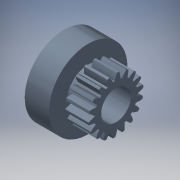
# Autodesk Inventor part: Clutch Gear
Saved by Autodesk Inventor 2019 Beta2 (Build 230110000, 110) ContinuousBuild 0
## iProperties
Created: 2012-08-06
Part Number: Clutch Gear
Material: Stainless Steel, 440C
Document SubType Name: Modeling
Designer: John
Density: 7.75 g/cm^3
Mass: 13.9161 g
Surface Area: 27.6405 cm^2
Volume: 1.79562 cm^3
Appearance: Steel Blue
Author: John
Autodesk Inventor part; units mm, degrees
ref_plane "YZ Plane" through (0, 0, 0) normal (1, 0, 0) x (0, 1, 0)
ref_plane "XZ Plane" through (0, 0, 0) normal (0, 1, 0) x (-1, 0, 0)
ref_plane "XY Plane" through (0, 0, 0) normal (0, 0, 1) x (1, 0, 0)
sketch "Sketch1" plane through (0, 0, 0) normal (1, 0, 0) x (0, 1, 0)
  circle A0 centre (0, 0) radius 12.5095
  dimension "d0" = 25.019
  constraints: 1 centre point, 1 coincident
  measures "d0" diameter of A0
extrude "Extrusion1" add sketch "Sketch1" along normal blind 7.747
sketch "Sketch3" plane through (7.747, 0, 0) normal (1, 0, 0) x (0, 0, -1)
  circle A0 centre (0, 0) radius 12.5095 projected
  circle A1 centre (0, 0) radius 8.763
  dimension "d3" = 17.526
  constraints: 1 centre point, 1 coincident
  measures "d3" diameter of A1
extrude "Extrusion2" add sketch "Sketch3" along normal blind 8.89 contours A1
sketch "Sketch4" plane through (7.747, 0, 0) normal (1, 0, 0) x (0, 0, -1)
  circle A0 centre (0, 0) radius 8.763 projected
  circle A1 centre (0, 0) radius 6.7818
  dimension "d26" = 6.7818
  constraints: 1 centre point
  measures "d26" radius of A1
extrude "Extrusion3" cut sketch "Sketch4" along normal blind 1.397
sketch "Sketch5" plane through (16.637, 0, 0) normal (1, 0, 0) x (0, 0, -1)
  circle A0 centre (0, 0) radius 8.763 projected
hole "Hole1" at (16.637, 0, 0) direction (-1, 0, 0) diameter 9.525 end through all
sketch "Sketch6" plane through (0, 0, 0) normal (-1, 0, 0) x (0, 0, 1)
  circle A0 centre (0, 0) radius 4.7625 projected
hole "Hole2" at (0, 0, 0) direction (1, 0, 0) diameter 23.114 depth 6.8072
sketch "Sketch7" plane through (16.637, 0, 0) normal (1, 0, 0) x (0, 0, -1)
  circle A0 centre (0, 0) radius 8.763 projected
  arc A1 (6.3049, -2.5147) -> (8.3872, -2.5234) centre (7.3744, 4.2693) ccw
  arc A2 (8.3872, -2.5234) -> (8.5753, -1.7828) centre (0, 0) ccw
  arc A3 (8.5753, -1.7828) -> (6.741, -0.7972) centre (4.445, -7.2699) ccw
  arc A4 (6.741, -0.7972) -> (6.7848, -0.2067) centre (0, 0) ccw
  arc A5 (6.7848, -0.2067) -> (8.7445, 0.4974) centre (5.4695, 6.534) ccw
  arc A6 (8.7445, 0.4974) -> (8.6679, 1.2576) centre (0, 0) ccw
  arc A7 (8.6679, 1.2576) -> (6.6071, 1.5564) centre (6.6633, -5.3112) ccw
  arc A8 (6.6071, 1.5564) -> (6.4463, 2.1263) centre (0, 0) ccw
  arc A9 (6.4463, 2.1263) -> (8.047, 3.4581) centre (2.9049, 8.0107) ccw
  arc A10 (8.047, 3.4581) -> (7.715, 4.1463) centre (0, 0) ccw
  arc A11 (7.715, 4.1463) -> (5.6763, 3.7223) centre (8.078, -2.7119) ccw
  arc A12 (5.6763, 3.7223) -> (5.3303, 4.2029) centre (0, 0) ccw
  arc A13 (5.3303, 4.2029) -> (6.379, 6.0018) centre (-0.0101, 8.5211) ccw
  arc A14 (6.379, 6.0018) -> (5.8316, 6.535) centre (0, 0) ccw
  arc A15 (5.8316, 6.535) -> (4.0609, 5.4392) centre (8.5184, 0.2145) ccw
  arc A16 (4.0609, 5.4392) -> (3.5714, 5.7725) centre (0, 0) ccw
  arc A17 (3.5714, 5.7725) -> (3.9415, 7.8216) centre (-2.9239, 8.0037) ccw
  arc A18 (3.9415, 7.8216) -> (3.2448, 8.1354) centre (0, 0) ccw
  arc A19 (3.2448, 8.1354) -> (1.9557, 6.5001) centre (7.9313, 3.115) ccw
  arc A20 (1.9557, 6.5001) -> (1.3817, 6.6458) centre (0, 0) ccw
  arc A21 (1.3817, 6.6458) -> (1.0287, 8.698) centre (-5.485, 6.521) ccw
  arc A22 (1.0287, 8.698) -> (0.2667, 8.7546) centre (0, 0) ccw
  arc A23 (0.2667, 8.7546) -> (-0.3854, 6.777) centre (6.3876, 5.6398) ccw
  arc A24 (-0.3854, 6.777) -> (-0.9746, 6.7176) centre (0, 0) ccw
  arc A25 (-0.9746, 6.7176) -> (-2.0083, 8.5253) centre (-7.3845, 4.2518) ccw
  arc A26 (-2.0083, 8.5253) -> (-2.7436, 8.3178) centre (0, 0) ccw
  arc A27 (-2.7436, 8.3178) -> (-2.6801, 6.2364) centre (4.0734, 7.4844) ccw
  arc A28 (-2.6801, 6.2364) -> (-3.2134, 5.9791) centre (0, 0) ccw
  arc A29 (-3.2134, 5.9791) -> (-4.803, 7.3243) centre (-8.3934, 1.4697) ccw
  arc A30 (-4.803, 7.3243) -> (-5.423, 6.8778) centre (0, 0) ccw
  arc A31 (-5.423, 6.8778) -> (-4.6514, 4.9437) centre (1.268, 8.4262) ccw
  arc A32 (-4.6514, 4.9437) -> (-5.0646, 4.5195) centre (0, 0) ccw
  arc A33 (-5.0646, 4.5195) -> (-7.0184, 5.2399) centre (-8.3899, -1.4896) ccw
  arc A34 (-7.0184, 5.2399) -> (-7.4483, 4.6082) centre (0, 0) ccw
  arc A35 (-7.4483, 4.6082) -> (-6.0618, 3.0547) centre (-1.6904, 8.3517) ccw
  arc A36 (-6.0618, 3.0547) -> (-6.3049, 2.5147) centre (0, 0) ccw
  arc A37 (-6.3049, 2.5147) -> (-8.3872, 2.5234) centre (-7.3744, -4.2693) ccw
  arc A38 (-8.3872, 2.5234) -> (-8.5753, 1.7828) centre (0, 0) ccw
  arc A39 (-8.5753, 1.7828) -> (-6.741, 0.7972) centre (-4.445, 7.2699) ccw
  arc A40 (-6.741, 0.7972) -> (-6.7848, 0.2067) centre (0, 0) ccw
  arc A41 (-6.7848, 0.2067) -> (-8.7445, -0.4974) centre (-5.4695, -6.534) ccw
  arc A42 (-8.7445, -0.4974) -> (-8.6679, -1.2576) centre (0, 0) ccw
  arc A43 (-8.6679, -1.2576) -> (-6.6071, -1.5564) centre (-6.6633, 5.3112) ccw
  arc A44 (-6.6071, -1.5564) -> (-6.4463, -2.1263) centre (0, 0) ccw
  arc A45 (-6.4463, -2.1263) -> (-8.047, -3.4581) centre (-2.9049, -8.0107) ccw
  arc A46 (-8.047, -3.4581) -> (-7.715, -4.1463) centre (0, 0) ccw
  arc A47 (-7.715, -4.1463) -> (-5.6763, -3.7223) centre (-8.078, 2.7119) ccw
  arc A48 (-5.6763, -3.7223) -> (-5.3303, -4.2029) centre (0, 0) ccw
  arc A49 (-5.3303, -4.2029) -> (-6.379, -6.0018) centre (0.0101, -8.5211) ccw
  arc A50 (-6.379, -6.0018) -> (-5.8316, -6.535) centre (0, 0) ccw
  arc A51 (-5.8316, -6.535) -> (-4.0609, -5.4392) centre (-8.5184, -0.2145) ccw
  arc A52 (-4.0609, -5.4392) -> (-3.5714, -5.7725) centre (0, 0) ccw
  arc A53 (-3.5714, -5.7725) -> (-3.9415, -7.8216) centre (2.9239, -8.0037) ccw
  arc A54 (-3.9415, -7.8216) -> (-3.2448, -8.1354) centre (0, 0) ccw
  arc A55 (-3.2448, -8.1354) -> (-1.9557, -6.5001) centre (-7.9313, -3.115) ccw
  arc A56 (-1.9557, -6.5001) -> (-1.3817, -6.6458) centre (0, 0) ccw
  arc A57 (-1.3817, -6.6458) -> (-1.0287, -8.698) centre (5.485, -6.521) ccw
  arc A58 (-1.0287, -8.698) -> (-0.2667, -8.7546) centre (0, 0) ccw
  arc A59 (-0.2667, -8.7546) -> (0.3854, -6.777) centre (-6.3876, -5.6398) ccw
  arc A60 (0.3854, -6.777) -> (0.9746, -6.7176) centre (0, 0) ccw
  arc A61 (0.9746, -6.7176) -> (2.0083, -8.5253) centre (7.3845, -4.2518) ccw
  arc A62 (2.0083, -8.5253) -> (2.7436, -8.3178) centre (0, 0) ccw
  arc A63 (2.7436, -8.3178) -> (2.6801, -6.2364) centre (-4.0734, -7.4844) ccw
  arc A64 (2.6801, -6.2364) -> (3.2134, -5.9791) centre (0, 0) ccw
  arc A65 (3.2134, -5.9791) -> (4.803, -7.3243) centre (8.3934, -1.4697) ccw
  arc A66 (4.803, -7.3243) -> (5.423, -6.8778) centre (0, 0) ccw
  arc A67 (5.423, -6.8778) -> (4.6514, -4.9437) centre (-1.268, -8.4262) ccw
  arc A68 (4.6514, -4.9437) -> (5.0646, -4.5195) centre (0, 0) ccw
  arc A69 (5.0646, -4.5195) -> (7.0184, -5.2399) centre (8.3899, 1.4896) ccw
  arc A70 (7.0184, -5.2399) -> (7.4483, -4.6082) centre (0, 0) ccw
  arc A71 (7.4483, -4.6082) -> (6.0618, -3.0547) centre (1.6904, -8.3517) ccw
  arc A72 (6.0618, -3.0547) -> (6.3049, -2.5147) centre (0, 0) ccw
  constraints: 144 point on circle, 72 centre point
extrude "Extrusion4" cut sketch "Sketch7" against normal up to surface (7.493 mm away)
body "Solid1"
